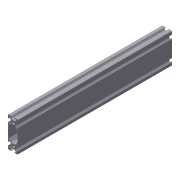
# Autodesk Inventor part: Bosch 20x60
Saved by Autodesk Inventor 2013 (Build 170138000, 138)
## iProperties
Created: 2011-07-21
Part Number: Bosch 20x60
Material: Aluminum-6061
Document SubType Name: Modeling
Designer: Dan Niemitalo
Mass: 296.662 g
Surface Area: 1227.79 cm^2
Volume: 109.469 cm^3
Density: 2.71 g/cm^3
Author: Dan Niemitalo
Autodesk Inventor part; units mm, degrees
ref_plane "YZ Plane" through (0, 0, 0) normal (1, 0, 0) x (0, 1, 0)
ref_plane "XZ Plane" through (0, 0, 0) normal (0, 1, 0) x (-1, 0, 0)
ref_plane "XY Plane" through (0, 0, 0) normal (0, 0, 1) x (1, 0, 0)
sketch "2060" plane through (0, 0, 0) normal (0, 0, 1) x (1, 0, 0)
  line L0 (-1.4693, -31.5636) -> (-0.9592, -32.4471)
  arc A0 (-0.9592, -32.6471) -> (-0.9592, -32.4471) centre (-1.1324, -32.5471) ccw
  line L1 (-0.9592, -32.6471) -> (-1.4693, -33.5306)
  arc A1 (-1.4693, -33.5306) -> (-1.4961, -33.6306) centre (-1.2961, -33.6306) ccw
  line L2 (-1.4961, -33.6306) -> (-1.4961, -35.6543)
  line L3 (0.6358, -33.8094) -> (0.0893, -34.461)
  arc A2 (0.0893, -34.461) -> (1.169, -35.5393) centre (3.0789, -32.5471) ccw
  line L4 (1.169, -35.5393) -> (1.8208, -34.9924)
  arc A3 (2.1254, -37.0471) -> (2.2254, -37.0203) centre (2.1254, -36.8471) ccw
  line L5 (2.2254, -37.0203) -> (2.9789, -36.5852)
  arc A4 (3.1789, -36.5852) -> (2.9789, -36.5852) centre (3.0789, -36.7584) ccw
  line L6 (3.1789, -36.5852) -> (3.9325, -37.0203)
  arc A5 (3.9325, -37.0203) -> (4.0325, -37.0471) centre (4.0325, -36.8471) ccw
  line L7 (4.0325, -37.0471) -> (6.3112, -37.0471)
  line L8 (7.6539, -35.6543) -> (7.6539, -33.6306)
  arc A6 (4.9928, -35.5368) -> (6.0711, -34.457) centre (3.0789, -32.5471) ccw
  line L9 (6.0711, -34.457) -> (5.5242, -33.8053)
  line L10 (4.3413, -34.9902) -> (4.9928, -35.5368)
  arc A7 (7.6539, -35.6543) -> (7.8004, -36.0079) centre (8.1539, -35.6543) ccw
  line L11 (4.9889, -29.5549) -> (4.3371, -30.1018)
  line L12 (1.8166, -30.1039) -> (1.165, -29.5575)
  arc A8 (6.0686, -30.6332) -> (4.9889, -29.5549) centre (3.0789, -32.5471) ccw
  arc A9 (1.165, -29.5575) -> (0.0868, -30.6372) centre (3.0789, -32.5471) ccw
  line L13 (0.0868, -30.6372) -> (0.6336, -31.2889)
  line L14 (5.5242, -31.2889) -> (6.0686, -30.6332)
  arc A10 (0.6336, -31.2889) -> (0.6358, -33.8094) centre (3.0789, -32.5471) ccw
  arc A11 (5.5242, -33.8053) -> (5.5242, -31.2889) centre (3.0789, -32.5471) ccw
  arc A12 (1.8208, -34.9924) -> (4.3413, -34.9902) centre (3.0789, -32.5471) ccw
  arc A13 (4.3371, -30.1018) -> (1.8166, -30.1039) centre (3.0789, -32.5471) ccw
  line L15 (7.6539, -31.4636) -> (7.6539, -29.4399)
  line L16 (7.1171, -32.4471) -> (7.6271, -31.5636)
  arc A14 (7.1171, -32.4471) -> (7.1171, -32.6471) centre (7.2903, -32.5471) ccw
  arc A15 (7.6539, -33.6306) -> (7.6271, -33.5306) centre (7.4539, -33.6306) ccw
  line L17 (7.6271, -33.5306) -> (7.1171, -32.6471)
  arc A16 (7.6271, -31.5636) -> (7.6539, -31.4636) centre (7.4539, -31.4636) ccw
  arc A17 (2.9789, -28.509) -> (3.1789, -28.509) centre (3.0789, -28.3358) ccw
  line L18 (3.1789, -28.509) -> (3.9325, -28.0739)
  line L19 (2.2254, -28.0739) -> (2.9789, -28.509)
  arc A18 (7.8004, -29.0863) -> (7.6539, -29.4399) centre (8.1539, -29.4399) ccw
  line L20 (7.8004, -29.0863) -> (10.1932, -26.6935)
  arc A19 (11.5789, -29.0471) -> (12.0789, -29.5471) centre (12.0789, -29.0471) ccw
  arc A20 (12.3789, -29.5471) -> (12.5789, -29.3471) centre (12.3789, -29.3471) ccw
  line L21 (12.5789, -29.3471) -> (12.5789, -29.2471)
  arc A21 (12.7789, -29.0471) -> (12.5789, -29.2471) centre (12.7789, -29.2471) ccw
  line L22 (12.7789, -29.0471) -> (12.8789, -29.0471)
  line L23 (11.5789, -27.0471) -> (11.5789, -29.0471)
  arc A22 (12.8789, -29.0471) -> (13.0789, -28.8471) centre (12.8789, -28.8471) ccw
  line L24 (12.0789, -29.5471) -> (12.3789, -29.5471)
  arc A23 (-5.4211, -36.0471) -> (-5.9211, -35.5471) centre (-5.9211, -36.0471) ccw
  line L25 (-5.9211, -35.5471) -> (-6.2211, -35.5471)
  line L26 (-6.6211, -36.0971) -> (-6.7211, -36.0971)
  line L27 (-6.4211, -35.7471) -> (-6.4211, -35.8971)
  arc A24 (-6.6211, -36.0971) -> (-6.4211, -35.8971) centre (-6.6211, -35.8971) ccw
  arc A25 (-6.7211, -36.0971) -> (-6.9211, -36.2971) centre (-6.7211, -36.2971) ccw
  arc A26 (-6.2211, -35.5471) -> (-6.4211, -35.7471) centre (-6.2211, -35.7471) ccw
  arc A27 (-1.4961, -31.4636) -> (-1.4693, -31.5636) centre (-1.2961, -31.4636) ccw
  line L28 (-1.4961, -29.4399) -> (-1.4961, -31.4636)
  arc A28 (-1.4961, -29.4399) -> (-1.6425, -29.0863) centre (-1.9961, -29.4399) ccw
  line L29 (-6.2211, -29.5471) -> (-5.9211, -29.5471)
  arc A29 (-5.9211, -29.5471) -> (-5.4211, -29.0471) centre (-5.9211, -29.0471) ccw
  arc A30 (-6.4211, -29.3471) -> (-6.2211, -29.5471) centre (-6.2211, -29.3471) ccw
  line L30 (-6.4211, -29.1971) -> (-6.4211, -29.3471)
  arc A31 (-6.4211, -29.1971) -> (-6.6211, -28.9971) centre (-6.6211, -29.1971) ccw
  line L31 (-6.7211, -28.9971) -> (-6.6211, -28.9971)
  arc A32 (-6.9211, -28.7971) -> (-6.7211, -28.9971) centre (-6.7211, -28.7971) ccw
  line L32 (-4.9211, -26.5471) -> (-4.3888, -26.5471)
  line L33 (-4.0353, -26.6935) -> (-1.6425, -29.0863)
  line L34 (-5.4211, -29.0471) -> (-5.4211, -27.0471)
  arc A33 (-4.0353, -26.6935) -> (-4.3888, -26.5471) centre (-4.3888, -27.0471) ccw
  line L35 (11.5789, 3.9087) -> (11.5789, 1.9587)
  arc A34 (11.0789, 1.4587) -> (11.5789, 1.9587) centre (11.0789, 1.9587) ccw
  line L36 (11.0789, 1.4587) -> (10.3467, 1.4587)
  arc A35 (9.9932, 1.6051) -> (10.3467, 1.4587) centre (10.3467, 1.9587) ccw
  line L37 (11.5789, -2.102) -> (6.6647, 2.8122)
  line L38 (9.9932, 1.6051) -> (7.8004, 3.7979)
  arc A36 (6.6647, 2.8122) -> (6.3112, 2.9587) centre (6.3112, 2.4587) ccw
  line L39 (6.3112, 2.9587) -> (4.0325, 2.9587)
  arc A37 (3.9325, 2.9855) -> (4.0325, 2.9587) centre (4.0325, 3.1587) ccw
  line L40 (3.9325, 2.9855) -> (3.1789, 3.4206)
  arc A38 (3.1789, 3.4206) -> (2.9789, 3.4206) centre (3.0789, 3.2474) ccw
  line L41 (2.9789, 3.4206) -> (2.2254, 2.9855)
  arc A39 (2.1254, 2.9587) -> (2.2254, 2.9855) centre (2.1254, 3.1587) ccw
  arc A40 (12.0789, 4.4087) -> (11.5789, 3.9087) centre (12.0789, 3.9087) ccw
  line L42 (12.3789, 4.4087) -> (12.0789, 4.4087)
  line L43 (12.8789, 3.9087) -> (12.7789, 3.9087)
  line L44 (12.5789, 4.1087) -> (12.5789, 4.2087)
  arc A41 (12.5789, 4.1087) -> (12.7789, 3.9087) centre (12.7789, 4.1087) ccw
  arc A42 (12.5789, 4.2087) -> (12.3789, 4.4087) centre (12.3789, 4.2087) ccw
  arc A43 (13.0789, 3.7087) -> (12.8789, 3.9087) centre (12.8789, 3.7087) ccw
  line L45 (4.3371, 5.0134) -> (4.966, 4.511)
  arc A44 (4.966, 4.511) -> (6.0267, 5.5716) centre (3.0789, 7.4587) ccw
  line L46 (6.0267, 5.5716) -> (5.5242, 6.2005)
  arc A45 (7.6539, 4.1515) -> (7.8004, 3.7979) centre (8.1539, 4.1515) ccw
  line L47 (7.6539, 4.1515) -> (7.6539, 6.6301)
  line L48 (-5.4211, 1.9587) -> (-5.4211, 3.9087)
  arc A46 (-5.4211, 1.9587) -> (-4.9211, 1.4587) centre (-4.9211, 1.9587) ccw
  line L49 (-4.1888, 1.4587) -> (-4.9211, 1.4587)
  arc A47 (-4.1888, 1.4587) -> (-3.8353, 1.6051) centre (-4.1888, 1.9587) ccw
  arc A48 (-1.6425, 3.7979) -> (-1.4961, 4.1515) centre (-1.9961, 4.1515) ccw
  line L50 (-1.6425, 3.7979) -> (-3.8353, 1.6051)
  arc A49 (-0.1533, 2.9587) -> (-0.5068, 2.8122) centre (-0.1533, 2.4587) ccw
  line L51 (-0.5068, 2.8122) -> (-5.4211, -2.102)
  arc A50 (-4.9211, -26.5471) -> (-5.4211, -27.0471) centre (-4.9211, -27.0471) ccw
  arc A51 (-0.5068, -27.9006) -> (-0.1533, -28.0471) centre (-0.1533, -27.5471) ccw
  line L52 (-0.1533, -28.0471) -> (2.1254, -28.0471)
  arc A52 (2.2254, -28.0739) -> (2.1254, -28.0471) centre (2.1254, -28.2471) ccw
  line L53 (-5.4211, -22.9864) -> (-0.5068, -27.9006)
  arc A53 (4.0325, -28.0471) -> (3.9325, -28.0739) centre (4.0325, -28.2471) ccw
  line L54 (4.0325, -28.0471) -> (6.3112, -28.0471)
  arc A54 (6.3112, -28.0471) -> (6.6647, -27.9006) centre (6.3112, -27.5471) ccw
  arc A55 (10.5467, -26.5471) -> (10.1932, -26.6935) centre (10.5467, -27.0471) ccw
  line L55 (10.5467, -26.5471) -> (11.0789, -26.5471)
  arc A56 (11.5789, -27.0471) -> (11.0789, -26.5471) centre (11.0789, -27.0471) ccw
  line L56 (6.6647, -27.9006) -> (11.5789, -22.9864)
  line L57 (-6.9211, 3.7087) -> (-6.9211, -28.7971)
  line L58 (13.0789, -28.8471) -> (13.0789, 3.7087)
  line L59 (11.5789, -22.9864) -> (11.5789, -2.102)
  line L60 (-5.4211, -2.102) -> (-5.4211, -22.9864)
  arc A57 (-6.7211, 3.9087) -> (-6.9211, 3.7087) centre (-6.7211, 3.7087) ccw
  line L61 (-6.6211, 3.9087) -> (-6.7211, 3.9087)
  arc A58 (-6.6211, 3.9087) -> (-6.4211, 4.1087) centre (-6.6211, 4.1087) ccw
  arc A59 (-5.4211, 3.9087) -> (-5.9211, 4.4087) centre (-5.9211, 3.9087) ccw
  line L62 (-5.9211, 4.4087) -> (-6.2211, 4.4087)
  arc A60 (-6.2211, 4.4087) -> (-6.4211, 4.2087) centre (-6.2211, 4.2087) ccw
  line L63 (-6.4211, 4.2087) -> (-6.4211, 4.1087)
  line L64 (5.5242, 8.7169) -> (6.0267, 9.3457)
  line L65 (4.966, 10.4064) -> (4.3371, 9.904)
  arc A61 (6.0267, 9.3457) -> (4.966, 10.4064) centre (3.0789, 7.4587) ccw
  arc A62 (11.5789, 10.9087) -> (12.0789, 10.4087) centre (12.0789, 10.9087) ccw
  line L66 (12.0789, 10.4087) -> (12.3789, 10.4087)
  line L67 (12.7789, 10.9087) -> (12.8789, 10.9087)
  line L68 (12.5789, 10.6087) -> (12.5789, 10.7087)
  arc A63 (12.7789, 10.9087) -> (12.5789, 10.7087) centre (12.7789, 10.7087) ccw
  arc A64 (12.3789, 10.4087) -> (12.5789, 10.6087) centre (12.3789, 10.6087) ccw
  arc A65 (12.8789, 10.9087) -> (13.0789, 11.1087) centre (12.8789, 11.1087) ccw
  arc A66 (5.5242, 6.2005) -> (5.5242, 8.7169) centre (3.0789, 7.4587) ccw
  arc A67 (1.8208, 5.0134) -> (4.3371, 5.0134) centre (3.0789, 7.4587) ccw
  line L69 (1.1919, 4.511) -> (1.8208, 5.0134)
  line L70 (2.1254, 2.9587) -> (-0.1533, 2.9587)
  arc A68 (0.1312, 5.5716) -> (1.1919, 4.511) centre (3.0789, 7.4587) ccw
  arc A69 (4.3371, 9.904) -> (1.8208, 9.904) centre (3.0789, 7.4587) ccw
  line L71 (0.6336, 6.2005) -> (0.1312, 5.5716)
  arc A70 (0.6336, 8.7169) -> (0.6336, 6.2005) centre (3.0789, 7.4587) ccw
  line L72 (1.8208, 9.904) -> (1.1919, 10.4064)
  line L73 (0.1312, 9.3457) -> (0.6336, 8.7169)
  arc A71 (1.1919, 10.4064) -> (0.1312, 9.3457) centre (3.0789, 7.4587) ccw
  arc A72 (7.6539, 6.6301) -> (7.6271, 6.7301) centre (7.4539, 6.6301) ccw
  line L74 (7.6271, 6.7301) -> (7.2209, 7.4337)
  arc A73 (7.2209, 7.6337) -> (7.2209, 7.4337) centre (7.3941, 7.5337) ccw
  line L75 (7.2209, 7.6337) -> (7.6271, 8.3373)
  arc A74 (7.6271, 8.3373) -> (7.6539, 8.4373) centre (7.4539, 8.4373) ccw
  line L76 (7.6539, 8.4373) -> (7.6539, 10.7659)
  arc A75 (6.3112, 11.9529) -> (6.6647, 12.0994) centre (6.3112, 12.4529) ccw
  arc A76 (-1.4961, 10.7659) -> (-1.6425, 11.1195) centre (-1.9961, 10.7659) ccw
  line L77 (-1.4961, 10.7659) -> (-1.4961, 8.4373)
  line L78 (6.3112, 11.9529) -> (4.0325, 11.9529)
  arc A77 (4.0325, 11.9529) -> (3.9325, 11.9261) centre (4.0325, 11.7529) ccw
  line L79 (3.9325, 11.9261) -> (3.1381, 11.4675)
  arc A78 (3.0197, 11.4675) -> (3.1381, 11.4675) centre (3.0789, 11.57) ccw
  arc A79 (2.2254, 11.9261) -> (2.1254, 11.9529) centre (2.1254, 11.7529) ccw
  line L80 (3.0197, 11.4675) -> (2.2254, 11.9261)
  line L81 (2.1254, 11.9529) -> (-0.1533, 11.9529)
  line L82 (-6.7211, 10.9087) -> (-6.6211, 10.9087)
  arc A80 (-6.4211, 10.7087) -> (-6.6211, 10.9087) centre (-6.6211, 10.7087) ccw
  line L83 (-6.4211, 10.7087) -> (-6.4211, 10.6087)
  line L84 (-6.2211, 10.4087) -> (-5.9211, 10.4087)
  arc A81 (-5.9211, 10.4087) -> (-5.4211, 10.9087) centre (-5.9211, 10.9087) ccw
  arc A82 (-6.4211, 10.6087) -> (-6.2211, 10.4087) centre (-6.2211, 10.6087) ccw
  arc A83 (-1.4961, 8.4373) -> (-1.4693, 8.3373) centre (-1.2961, 8.4373) ccw
  line L85 (-1.4693, 8.3373) -> (-1.063, 7.6337)
  arc A84 (-1.063, 7.4337) -> (-1.063, 7.6337) centre (-1.2363, 7.5337) ccw
  line L86 (-1.063, 7.4337) -> (-1.4693, 6.7301)
  arc A85 (-1.4693, 6.7301) -> (-1.4961, 6.6301) centre (-1.2961, 6.6301) ccw
  line L87 (-1.4961, 6.6301) -> (-1.4961, 4.1515)
  line L88 (9.0789, 15.4529) -> (9.0789, 14.7207)
  arc A86 (8.9325, 14.3671) -> (9.0789, 14.7207) centre (8.5789, 14.7207) ccw
  line L89 (8.9325, 14.3671) -> (6.6647, 12.0994)
  arc A87 (10.3467, 13.4587) -> (9.9932, 13.3122) centre (10.3467, 12.9587) ccw
  arc A88 (11.5789, 12.9587) -> (11.0789, 13.4587) centre (11.0789, 12.9587) ccw
  line L90 (7.8004, 11.1195) -> (9.9932, 13.3122)
  arc A89 (7.8004, 11.1195) -> (7.6539, 10.7659) centre (8.1539, 10.7659) ccw
  line L91 (13.0789, 11.1087) -> (13.0789, 15.9529)
  line L92 (11.5789, 12.9587) -> (11.5789, 10.9087)
  line L93 (10.3467, 13.4587) -> (11.0789, 13.4587)
  arc A90 (9.0789, 15.4529) -> (8.5789, 15.9529) centre (8.5789, 15.4529) ccw
  arc A91 (13.0789, 15.9529) -> (11.5789, 17.4529) centre (11.5789, 15.9529) ccw
  line L94 (11.5789, 17.4529) -> (6.8289, 17.4529)
  line L95 (6.5789, 15.9529) -> (8.5789, 15.9529)
  arc A92 (6.0789, 16.4529) -> (6.5789, 15.9529) centre (6.5789, 16.4529) ccw
  line L96 (6.6289, 17.2529) -> (6.6289, 17.1529)
  line L97 (6.0789, 16.7529) -> (6.0789, 16.4529)
  arc A93 (6.4289, 16.9529) -> (6.6289, 17.1529) centre (6.4289, 17.1529) ccw
  arc A94 (6.8289, 17.4529) -> (6.6289, 17.2529) centre (6.8289, 17.2529) ccw
  arc A95 (6.2789, 16.9529) -> (6.0789, 16.7529) centre (6.2789, 16.7529) ccw
  line L98 (6.4289, 16.9529) -> (6.2789, 16.9529)
  arc A96 (-0.4211, 15.9529) -> (0.0789, 16.4529) centre (-0.4211, 16.4529) ccw
  line L99 (-0.4711, 17.1529) -> (-0.4711, 17.2529)
  line L100 (-0.1211, 16.9529) -> (-0.2711, 16.9529)
  line L101 (0.0789, 16.4529) -> (0.0789, 16.7529)
  arc A97 (-0.4711, 17.1529) -> (-0.2711, 16.9529) centre (-0.2711, 17.1529) ccw
  arc A98 (-0.4711, 17.2529) -> (-0.6711, 17.4529) centre (-0.6711, 17.2529) ccw
  arc A99 (0.0789, 16.7529) -> (-0.1211, 16.9529) centre (-0.1211, 16.7529) ccw
  line L102 (-2.4211, 15.9529) -> (-0.4211, 15.9529)
  line L103 (-4.9211, 13.4587) -> (-4.1888, 13.4587)
  arc A100 (-3.8353, 13.3122) -> (-4.1888, 13.4587) centre (-4.1888, 12.9587) ccw
  line L104 (-2.9211, 14.7207) -> (-2.9211, 15.4529)
  arc A101 (-2.9211, 14.7207) -> (-2.7746, 14.3671) centre (-2.4211, 14.7207) ccw
  arc A102 (-2.4211, 15.9529) -> (-2.9211, 15.4529) centre (-2.4211, 15.4529) ccw
  line L105 (-0.6711, 17.4529) -> (-5.4211, 17.4529)
  line L106 (-3.8353, 13.3122) -> (-1.6425, 11.1195)
  line L107 (-0.5068, 12.0994) -> (-2.7746, 14.3671)
  arc A103 (-0.5068, 12.0994) -> (-0.1533, 11.9529) centre (-0.1533, 12.4529) ccw
  arc A104 (-4.9211, 13.4587) -> (-5.4211, 12.9587) centre (-4.9211, 12.9587) ccw
  line L108 (-5.4211, 10.9087) -> (-5.4211, 12.9587)
  arc A105 (-6.9211, 11.1087) -> (-6.7211, 10.9087) centre (-6.7211, 11.1087) ccw
  line L109 (-6.9211, 15.9529) -> (-6.9211, 11.1087)
  arc A106 (-5.4211, 17.4529) -> (-6.9211, 15.9529) centre (-5.4211, 15.9529) ccw
  arc A107 (6.6647, -37.1935) -> (6.3112, -37.0471) centre (6.3112, -37.5471) ccw
  arc A108 (-2.9211, -40.5471) -> (-2.4211, -41.0471) centre (-2.4211, -40.5471) ccw
  line L110 (-2.9211, -40.5471) -> (-2.9211, -39.8149)
  arc A109 (-2.7746, -39.4613) -> (-2.9211, -39.8149) centre (-2.4211, -39.8149) ccw
  line L111 (-2.7746, -39.4613) -> (-0.5068, -37.1935)
  line L112 (-1.6425, -36.0079) -> (-4.0353, -38.4006)
  arc A110 (-1.6425, -36.0079) -> (-1.4961, -35.6543) centre (-1.9961, -35.6543) ccw
  arc A111 (-0.1533, -37.0471) -> (-0.5068, -37.1935) centre (-0.1533, -37.5471) ccw
  line L113 (-0.1533, -37.0471) -> (2.1254, -37.0471)
  line L114 (10.1932, -38.4006) -> (7.8004, -36.0079)
  line L115 (9.0789, -39.8149) -> (9.0789, -40.5471)
  arc A112 (9.0789, -39.8149) -> (8.9325, -39.4613) centre (8.5789, -39.8149) ccw
  line L116 (6.6647, -37.1935) -> (8.9325, -39.4613)
  arc A113 (10.1932, -38.4006) -> (10.5467, -38.5471) centre (10.5467, -38.0471) ccw
  line L117 (11.0789, -38.5471) -> (10.5467, -38.5471)
  arc A114 (11.0789, -38.5471) -> (11.5789, -38.0471) centre (11.0789, -38.0471) ccw
  line L118 (11.5789, -36.0471) -> (11.5789, -38.0471)
  arc A115 (12.0789, -35.5471) -> (11.5789, -36.0471) centre (12.0789, -36.0471) ccw
  line L119 (12.3789, -35.5471) -> (12.0789, -35.5471)
  arc A116 (12.5789, -35.7471) -> (12.3789, -35.5471) centre (12.3789, -35.7471) ccw
  line L120 (12.5789, -35.8471) -> (12.5789, -35.7471)
  arc A117 (12.5789, -35.8471) -> (12.7789, -36.0471) centre (12.7789, -35.8471) ccw
  line L121 (12.8789, -36.0471) -> (12.7789, -36.0471)
  arc A118 (13.0789, -36.2471) -> (12.8789, -36.0471) centre (12.8789, -36.2471) ccw
  line L122 (13.0789, -41.0471) -> (13.0789, -36.2471)
  arc A119 (-4.3888, -38.5471) -> (-4.0353, -38.4006) centre (-4.3888, -38.0471) ccw
  line L123 (-4.3888, -38.5471) -> (-4.9211, -38.5471)
  arc A120 (-6.9211, -41.0471) -> (-5.4211, -42.5471) centre (-5.4211, -41.0471) ccw
  arc A121 (-5.4211, -38.0471) -> (-4.9211, -38.5471) centre (-4.9211, -38.0471) ccw
  line L124 (-6.9211, -36.2971) -> (-6.9211, -41.0471)
  line L125 (-5.4211, -38.0471) -> (-5.4211, -36.0471)
  arc A122 (0.0789, -41.5471) -> (-0.4211, -41.0471) centre (-0.4211, -41.5471) ccw
  line L126 (0.0789, -41.8471) -> (0.0789, -41.5471)
  arc A123 (-0.1211, -42.0471) -> (0.0789, -41.8471) centre (-0.1211, -41.8471) ccw
  line L127 (-0.2711, -42.0471) -> (-0.1211, -42.0471)
  arc A124 (-0.2711, -42.0471) -> (-0.4711, -42.2471) centre (-0.2711, -42.2471) ccw
  line L128 (-0.4711, -42.3471) -> (-0.4711, -42.2471)
  arc A125 (-0.6711, -42.5471) -> (-0.4711, -42.3471) centre (-0.6711, -42.3471) ccw
  line L129 (-5.4211, -42.5471) -> (-0.6711, -42.5471)
  line L130 (-0.4211, -41.0471) -> (-2.4211, -41.0471)
  line L131 (6.6289, -42.2471) -> (6.6289, -42.3471)
  line L132 (6.2789, -42.0471) -> (6.4289, -42.0471)
  line L133 (6.0789, -41.5471) -> (6.0789, -41.8471)
  arc A126 (6.6289, -42.2471) -> (6.4289, -42.0471) centre (6.4289, -42.2471) ccw
  arc A127 (6.6289, -42.3471) -> (6.8289, -42.5471) centre (6.8289, -42.3471) ccw
  arc A128 (6.0789, -41.8471) -> (6.2789, -42.0471) centre (6.2789, -41.8471) ccw
  arc A129 (6.5789, -41.0471) -> (6.0789, -41.5471) centre (6.5789, -41.5471) ccw
  arc A130 (11.5789, -42.5471) -> (13.0789, -41.0471) centre (11.5789, -41.0471) ccw
  line L134 (6.8289, -42.5471) -> (11.5789, -42.5471)
  line L135 (8.5789, -41.0471) -> (6.5789, -41.0471)
  arc A131 (8.5789, -41.0471) -> (9.0789, -40.5471) centre (8.5789, -40.5471) ccw
  point P0 (3.0789, -12.5479)
sketch "Sketch1" plane through (0, 0, 0) normal (0, 0, 1) x (1, 0, 0)
  line L0 (-4.5482, -19.0194) -> (-4.0381, -19.9029)
  arc A0 (-4.0381, -20.1029) -> (-4.0381, -19.9029) centre (-4.2113, -20.0029) ccw
  line L1 (-4.0381, -20.1029) -> (-4.5482, -20.9864)
  arc A1 (-4.5482, -20.9864) -> (-4.575, -21.0864) centre (-4.375, -21.0864) ccw
  line L2 (-4.575, -21.0864) -> (-4.575, -23.1101)
  line L3 (-2.4431, -21.2652) -> (-2.9897, -21.9168)
  arc A2 (-2.9897, -21.9168) -> (-1.9099, -22.9951) centre (0, -20.0029) ccw
  line L4 (-1.9099, -22.9951) -> (-1.2582, -22.4482)
  arc A3 (-0.9536, -24.5029) -> (-0.8536, -24.4761) centre (-0.9536, -24.3029) ccw
  line L5 (-0.8536, -24.4761) -> (-0.1, -24.041)
  arc A4 (0.1, -24.041) -> (-0.1, -24.041) centre (0, -24.2142) ccw
  line L6 (0.1, -24.041) -> (0.8536, -24.4761)
  arc A5 (0.8536, -24.4761) -> (0.9536, -24.5029) centre (0.9536, -24.3029) ccw
  line L7 (0.9536, -24.5029) -> (3.2322, -24.5029)
  line L8 (4.575, -23.1101) -> (4.575, -21.0864)
  arc A6 (1.9139, -22.9926) -> (2.9922, -21.9128) centre (0, -20.0029) ccw
  line L9 (2.9922, -21.9128) -> (2.4453, -21.2611)
  line L10 (1.2623, -22.446) -> (1.9139, -22.9926)
  arc A7 (4.575, -23.1101) -> (4.7214, -23.4637) centre (5.075, -23.1101) ccw
  line L11 (1.9099, -17.0107) -> (1.2582, -17.5576)
  line L12 (-1.2623, -17.5597) -> (-1.9139, -17.0133)
  arc A8 (2.9896, -18.089) -> (1.9099, -17.0107) centre (0, -20.0029) ccw
  arc A9 (-1.9139, -17.0133) -> (-2.9922, -18.093) centre (0, -20.0029) ccw
  line L13 (-2.9922, -18.093) -> (-2.4453, -18.7447)
  line L14 (2.4453, -18.7447) -> (2.9896, -18.089)
  arc A10 (-2.4453, -18.7447) -> (-2.4431, -21.2652) centre (0, -20.0029) ccw
  arc A11 (2.4453, -21.2611) -> (2.4453, -18.7447) centre (0, -20.0029) ccw
  arc A12 (-1.2582, -22.4482) -> (1.2623, -22.446) centre (0, -20.0029) ccw
  arc A13 (1.2582, -17.5576) -> (-1.2623, -17.5597) centre (0, -20.0029) ccw
  line L15 (4.575, -18.9194) -> (4.575, -16.8957)
  line L16 (4.0381, -19.9029) -> (4.5482, -19.0194)
  arc A14 (4.0381, -19.9029) -> (4.0381, -20.1029) centre (4.2113, -20.0029) ccw
  arc A15 (4.575, -21.0864) -> (4.5482, -20.9864) centre (4.375, -21.0864) ccw
  line L17 (4.5482, -20.9864) -> (4.0381, -20.1029)
  arc A16 (4.5482, -19.0194) -> (4.575, -18.9194) centre (4.375, -18.9194) ccw
  arc A17 (-0.1, -15.9648) -> (0.1, -15.9648) centre (0, -15.7916) ccw
  line L18 (0.1, -15.9648) -> (0.8536, -15.5297)
  line L19 (-0.8536, -15.5297) -> (-0.1, -15.9648)
  arc A18 (4.7214, -16.5421) -> (4.575, -16.8957) centre (5.075, -16.8957) ccw
  line L20 (4.7214, -16.5421) -> (7.1142, -14.1493)
  arc A19 (8.5, -16.5029) -> (9, -17.0029) centre (9, -16.5029) ccw
  arc A20 (9.3, -17.0029) -> (9.5, -16.8029) centre (9.3, -16.8029) ccw
  line L21 (9.5, -16.8029) -> (9.5, -16.7029)
  arc A21 (9.7, -16.5029) -> (9.5, -16.7029) centre (9.7, -16.7029) ccw
  line L22 (9.7, -16.5029) -> (9.8, -16.5029)
  line L23 (8.5, -14.5029) -> (8.5, -16.5029)
  arc A22 (9.8, -16.5029) -> (10, -16.3029) centre (9.8, -16.3029) ccw
  line L24 (9, -17.0029) -> (9.3, -17.0029)
  arc A23 (-8.5, -23.5029) -> (-9, -23.0029) centre (-9, -23.5029) ccw
  line L25 (-9, -23.0029) -> (-9.3, -23.0029)
  line L26 (-9.7, -23.5529) -> (-9.8, -23.5529)
  line L27 (-9.5, -23.2029) -> (-9.5, -23.3529)
  arc A24 (-9.7, -23.5529) -> (-9.5, -23.3529) centre (-9.7, -23.3529) ccw
  arc A25 (-9.8, -23.5529) -> (-10, -23.7529) centre (-9.8, -23.7529) ccw
  arc A26 (-9.3, -23.0029) -> (-9.5, -23.2029) centre (-9.3, -23.2029) ccw
  arc A27 (-4.575, -18.9194) -> (-4.5482, -19.0194) centre (-4.375, -18.9194) ccw
  line L28 (-4.575, -16.8957) -> (-4.575, -18.9194)
  arc A28 (-4.575, -16.8957) -> (-4.7214, -16.5421) centre (-5.075, -16.8957) ccw
  line L29 (-9.3, -17.0029) -> (-9, -17.0029)
  arc A29 (-9, -17.0029) -> (-8.5, -16.5029) centre (-9, -16.5029) ccw
  arc A30 (-9.5, -16.8029) -> (-9.3, -17.0029) centre (-9.3, -16.8029) ccw
  line L30 (-9.5, -16.6529) -> (-9.5, -16.8029)
  arc A31 (-9.5, -16.6529) -> (-9.7, -16.4529) centre (-9.7, -16.6529) ccw
  line L31 (-9.8, -16.4529) -> (-9.7, -16.4529)
  arc A32 (-10, -16.2529) -> (-9.8, -16.4529) centre (-9.8, -16.2529) ccw
  line L32 (-8, -14.0029) -> (-7.4678, -14.0029)
  line L33 (-7.1142, -14.1493) -> (-4.7214, -16.5421)
  line L34 (-8.5, -16.5029) -> (-8.5, -14.5029)
  arc A33 (-7.1142, -14.1493) -> (-7.4678, -14.0029) centre (-7.4678, -14.5029) ccw
  line L35 (8.5, 16.4529) -> (8.5, 14.5029)
  arc A34 (8, 14.0029) -> (8.5, 14.5029) centre (8, 14.5029) ccw
  line L36 (8, 14.0029) -> (7.2678, 14.0029)
  arc A35 (6.9142, 14.1493) -> (7.2678, 14.0029) centre (7.2678, 14.5029) ccw
  line L37 (8.5, 10.4422) -> (3.5858, 15.3564)
  line L38 (6.9142, 14.1493) -> (4.7214, 16.3421)
  arc A36 (3.5858, 15.3564) -> (3.2322, 15.5029) centre (3.2322, 15.0029) ccw
  line L39 (3.2322, 15.5029) -> (0.9536, 15.5029)
  arc A37 (0.8536, 15.5297) -> (0.9536, 15.5029) centre (0.9536, 15.7029) ccw
  line L40 (0.8536, 15.5297) -> (0.1, 15.9648)
  arc A38 (0.1, 15.9648) -> (-0.1, 15.9648) centre (0, 15.7916) ccw
  line L41 (-0.1, 15.9648) -> (-0.8536, 15.5297)
  arc A39 (-0.9536, 15.5029) -> (-0.8536, 15.5297) centre (-0.9536, 15.7029) ccw
  arc A40 (9, 16.9529) -> (8.5, 16.4529) centre (9, 16.4529) ccw
  line L42 (9.3, 16.9529) -> (9, 16.9529)
  line L43 (9.8, 16.4529) -> (9.7, 16.4529)
  line L44 (9.5, 16.6529) -> (9.5, 16.7529)
  arc A41 (9.5, 16.6529) -> (9.7, 16.4529) centre (9.7, 16.6529) ccw
  arc A42 (9.5, 16.7529) -> (9.3, 16.9529) centre (9.3, 16.7529) ccw
  arc A43 (10, 16.2529) -> (9.8, 16.4529) centre (9.8, 16.2529) ccw
  line L45 (1.2582, 17.5576) -> (1.8871, 17.0552)
  arc A44 (1.8871, 17.0552) -> (2.9477, 18.1158) centre (0, 20.0029) ccw
  line L46 (2.9477, 18.1158) -> (2.4453, 18.7447)
  arc A45 (4.575, 16.6957) -> (4.7214, 16.3421) centre (5.075, 16.6957) ccw
  line L47 (4.575, 16.6957) -> (4.575, 19.1743)
  line L48 (-8.5, 14.5029) -> (-8.5, 16.4529)
  arc A46 (-8.5, 14.5029) -> (-8, 14.0029) centre (-8, 14.5029) ccw
  line L49 (-7.2678, 14.0029) -> (-8, 14.0029)
  arc A47 (-7.2678, 14.0029) -> (-6.9142, 14.1493) centre (-7.2678, 14.5029) ccw
  arc A48 (-4.7214, 16.3421) -> (-4.575, 16.6957) centre (-5.075, 16.6957) ccw
  line L50 (-4.7214, 16.3421) -> (-6.9142, 14.1493)
  arc A49 (-3.2322, 15.5029) -> (-3.5858, 15.3564) centre (-3.2322, 15.0029) ccw
  line L51 (-3.5858, 15.3564) -> (-8.5, 10.4422)
  arc A50 (-8, -14.0029) -> (-8.5, -14.5029) centre (-8, -14.5029) ccw
  arc A51 (-3.5858, -15.3564) -> (-3.2322, -15.5029) centre (-3.2322, -15.0029) ccw
  line L52 (-3.2322, -15.5029) -> (-0.9536, -15.5029)
  arc A52 (-0.8536, -15.5297) -> (-0.9536, -15.5029) centre (-0.9536, -15.7029) ccw
  line L53 (-8.5, -10.4422) -> (-3.5858, -15.3564)
  arc A53 (0.9536, -15.5029) -> (0.8536, -15.5297) centre (0.9536, -15.7029) ccw
  line L54 (0.9536, -15.5029) -> (3.2322, -15.5029)
  arc A54 (3.2322, -15.5029) -> (3.5858, -15.3564) centre (3.2322, -15.0029) ccw
  arc A55 (7.4678, -14.0029) -> (7.1142, -14.1493) centre (7.4678, -14.5029) ccw
  line L55 (7.4678, -14.0029) -> (8, -14.0029)
  arc A56 (8.5, -14.5029) -> (8, -14.0029) centre (8, -14.5029) ccw
  line L56 (3.5858, -15.3564) -> (8.5, -10.4422)
  line L57 (-10, 16.2529) -> (-10, -16.2529)
  line L58 (10, -16.3029) -> (10, 16.2529)
  line L59 (8.5, -10.4422) -> (8.5, 10.4422)
  line L60 (-8.5, 10.4422) -> (-8.5, -10.4422)
  arc A57 (-9.8, 16.4529) -> (-10, 16.2529) centre (-9.8, 16.2529) ccw
  line L61 (-9.7, 16.4529) -> (-9.8, 16.4529)
  arc A58 (-9.7, 16.4529) -> (-9.5, 16.6529) centre (-9.7, 16.6529) ccw
  arc A59 (-8.5, 16.4529) -> (-9, 16.9529) centre (-9, 16.4529) ccw
  line L62 (-9, 16.9529) -> (-9.3, 16.9529)
  arc A60 (-9.3, 16.9529) -> (-9.5, 16.7529) centre (-9.3, 16.7529) ccw
  line L63 (-9.5, 16.7529) -> (-9.5, 16.6529)
  line L64 (2.4453, 21.2611) -> (2.9477, 21.8899)
  line L65 (1.8871, 22.9506) -> (1.2582, 22.4482)
  arc A61 (2.9477, 21.8899) -> (1.8871, 22.9506) centre (0, 20.0029) ccw
  arc A62 (8.5, 23.4529) -> (9, 22.9529) centre (9, 23.4529) ccw
  line L66 (9, 22.9529) -> (9.3, 22.9529)
  line L67 (9.7, 23.4529) -> (9.8, 23.4529)
  line L68 (9.5, 23.1529) -> (9.5, 23.2529)
  arc A63 (9.7, 23.4529) -> (9.5, 23.2529) centre (9.7, 23.2529) ccw
  arc A64 (9.3, 22.9529) -> (9.5, 23.1529) centre (9.3, 23.1529) ccw
  arc A65 (9.8, 23.4529) -> (10, 23.6529) centre (9.8, 23.6529) ccw
  arc A66 (2.4453, 18.7447) -> (2.4453, 21.2611) centre (0, 20.0029) ccw
  arc A67 (-1.2582, 17.5576) -> (1.2582, 17.5576) centre (0, 20.0029) ccw
  line L69 (-1.8871, 17.0552) -> (-1.2582, 17.5576)
  line L70 (-0.9536, 15.5029) -> (-3.2322, 15.5029)
  arc A68 (-2.9477, 18.1158) -> (-1.8871, 17.0552) centre (0, 20.0029) ccw
  arc A69 (1.2582, 22.4482) -> (-1.2582, 22.4482) centre (0, 20.0029) ccw
  line L71 (-2.4453, 18.7447) -> (-2.9477, 18.1158)
  arc A70 (-2.4453, 21.2611) -> (-2.4453, 18.7447) centre (0, 20.0029) ccw
  line L72 (-1.2582, 22.4482) -> (-1.8871, 22.9506)
  line L73 (-2.9477, 21.8899) -> (-2.4453, 21.2611)
  arc A71 (-1.8871, 22.9506) -> (-2.9477, 21.8899) centre (0, 20.0029) ccw
  arc A72 (4.575, 19.1743) -> (4.5482, 19.2743) centre (4.375, 19.1743) ccw
  line L74 (4.5482, 19.2743) -> (4.142, 19.9779)
  arc A73 (4.142, 20.1779) -> (4.142, 19.9779) centre (4.3152, 20.0779) ccw
  line L75 (4.142, 20.1779) -> (4.5482, 20.8815)
  arc A74 (4.5482, 20.8815) -> (4.575, 20.9815) centre (4.375, 20.9815) ccw
  line L76 (4.575, 20.9815) -> (4.575, 23.3101)
  arc A75 (3.2322, 24.4971) -> (3.5858, 24.6436) centre (3.2322, 24.9971) ccw
  arc A76 (-4.575, 23.3101) -> (-4.7214, 23.6637) centre (-5.075, 23.3101) ccw
  line L77 (-4.575, 23.3101) -> (-4.575, 20.9815)
  line L78 (3.2322, 24.4971) -> (0.9536, 24.4971)
  arc A77 (0.9536, 24.4971) -> (0.8536, 24.4703) centre (0.9536, 24.2971) ccw
  line L79 (0.8536, 24.4703) -> (0.0592, 24.0117)
  arc A78 (-0.0592, 24.0117) -> (0.0592, 24.0117) centre (0, 24.1142) ccw
  arc A79 (-0.8536, 24.4703) -> (-0.9536, 24.4971) centre (-0.9536, 24.2971) ccw
  line L80 (-0.0592, 24.0117) -> (-0.8536, 24.4703)
  line L81 (-0.9536, 24.4971) -> (-3.2322, 24.4971)
  line L82 (-9.8, 23.4529) -> (-9.7, 23.4529)
  arc A80 (-9.5, 23.2529) -> (-9.7, 23.4529) centre (-9.7, 23.2529) ccw
  line L83 (-9.5, 23.2529) -> (-9.5, 23.1529)
  line L84 (-9.3, 22.9529) -> (-9, 22.9529)
  arc A81 (-9, 22.9529) -> (-8.5, 23.4529) centre (-9, 23.4529) ccw
  arc A82 (-9.5, 23.1529) -> (-9.3, 22.9529) centre (-9.3, 23.1529) ccw
  arc A83 (-4.575, 20.9815) -> (-4.5482, 20.8815) centre (-4.375, 20.9815) ccw
  line L85 (-4.5482, 20.8815) -> (-4.142, 20.1779)
  arc A84 (-4.142, 19.9779) -> (-4.142, 20.1779) centre (-4.3152, 20.0779) ccw
  line L86 (-4.142, 19.9779) -> (-4.5482, 19.2743)
  arc A85 (-4.5482, 19.2743) -> (-4.575, 19.1743) centre (-4.375, 19.1743) ccw
  line L87 (-4.575, 19.1743) -> (-4.575, 16.6957)
  line L88 (6, 27.9971) -> (6, 27.2649)
  arc A86 (5.8536, 26.9113) -> (6, 27.2649) centre (5.5, 27.2649) ccw
  line L89 (5.8536, 26.9113) -> (3.5858, 24.6436)
  arc A87 (7.2678, 26.0029) -> (6.9142, 25.8564) centre (7.2678, 25.5029) ccw
  arc A88 (8.5, 25.5029) -> (8, 26.0029) centre (8, 25.5029) ccw
  line L90 (4.7214, 23.6637) -> (6.9142, 25.8564)
  arc A89 (4.7214, 23.6637) -> (4.575, 23.3101) centre (5.075, 23.3101) ccw
  line L91 (10, 23.6529) -> (10, 28.4971)
  line L92 (8.5, 25.5029) -> (8.5, 23.4529)
  line L93 (7.2678, 26.0029) -> (8, 26.0029)
  arc A90 (6, 27.9971) -> (5.5, 28.4971) centre (5.5, 27.9971) ccw
  arc A91 (10, 28.4971) -> (8.5, 29.9971) centre (8.5, 28.4971) ccw
  line L94 (8.5, 29.9971) -> (3.75, 29.9971)
  line L95 (3.5, 28.4971) -> (5.5, 28.4971)
  arc A92 (3, 28.9971) -> (3.5, 28.4971) centre (3.5, 28.9971) ccw
  line L96 (3.55, 29.7971) -> (3.55, 29.6971)
  line L97 (3, 29.2971) -> (3, 28.9971)
  arc A93 (3.35, 29.4971) -> (3.55, 29.6971) centre (3.35, 29.6971) ccw
  arc A94 (3.75, 29.9971) -> (3.55, 29.7971) centre (3.75, 29.7971) ccw
  arc A95 (3.2, 29.4971) -> (3, 29.2971) centre (3.2, 29.2971) ccw
  line L98 (3.35, 29.4971) -> (3.2, 29.4971)
  arc A96 (-3.5, 28.4971) -> (-3, 28.9971) centre (-3.5, 28.9971) ccw
  line L99 (-3.55, 29.6971) -> (-3.55, 29.7971)
  line L100 (-3.2, 29.4971) -> (-3.35, 29.4971)
  line L101 (-3, 28.9971) -> (-3, 29.2971)
  arc A97 (-3.55, 29.6971) -> (-3.35, 29.4971) centre (-3.35, 29.6971) ccw
  arc A98 (-3.55, 29.7971) -> (-3.75, 29.9971) centre (-3.75, 29.7971) ccw
  arc A99 (-3, 29.2971) -> (-3.2, 29.4971) centre (-3.2, 29.2971) ccw
  line L102 (-5.5, 28.4971) -> (-3.5, 28.4971)
  line L103 (-8, 26.0029) -> (-7.2678, 26.0029)
  arc A100 (-6.9142, 25.8564) -> (-7.2678, 26.0029) centre (-7.2678, 25.5029) ccw
  line L104 (-6, 27.2649) -> (-6, 27.9971)
  arc A101 (-6, 27.2649) -> (-5.8536, 26.9113) centre (-5.5, 27.2649) ccw
  arc A102 (-5.5, 28.4971) -> (-6, 27.9971) centre (-5.5, 27.9971) ccw
  line L105 (-3.75, 29.9971) -> (-8.5, 29.9971)
  line L106 (-6.9142, 25.8564) -> (-4.7214, 23.6637)
  line L107 (-3.5858, 24.6436) -> (-5.8536, 26.9113)
  arc A103 (-3.5858, 24.6436) -> (-3.2322, 24.4971) centre (-3.2322, 24.9971) ccw
  arc A104 (-8, 26.0029) -> (-8.5, 25.5029) centre (-8, 25.5029) ccw
  line L108 (-8.5, 23.4529) -> (-8.5, 25.5029)
  arc A105 (-10, 23.6529) -> (-9.8, 23.4529) centre (-9.8, 23.6529) ccw
  line L109 (-10, 28.4971) -> (-10, 23.6529)
  arc A106 (-8.5, 29.9971) -> (-10, 28.4971) centre (-8.5, 28.4971) ccw
  arc A107 (3.5858, -24.6493) -> (3.2322, -24.5029) centre (3.2322, -25.0029) ccw
  arc A108 (-6, -28.0029) -> (-5.5, -28.5029) centre (-5.5, -28.0029) ccw
  line L110 (-6, -28.0029) -> (-6, -27.2707)
  arc A109 (-5.8536, -26.9171) -> (-6, -27.2707) centre (-5.5, -27.2707) ccw
  line L111 (-5.8536, -26.9171) -> (-3.5858, -24.6493)
  line L112 (-4.7214, -23.4637) -> (-7.1142, -25.8564)
  arc A110 (-4.7214, -23.4637) -> (-4.575, -23.1101) centre (-5.075, -23.1101) ccw
  arc A111 (-3.2322, -24.5029) -> (-3.5858, -24.6493) centre (-3.2322, -25.0029) ccw
  line L113 (-3.2322, -24.5029) -> (-0.9536, -24.5029)
  line L114 (7.1142, -25.8564) -> (4.7214, -23.4637)
  line L115 (6, -27.2707) -> (6, -28.0029)
  arc A112 (6, -27.2707) -> (5.8536, -26.9171) centre (5.5, -27.2707) ccw
  line L116 (3.5858, -24.6493) -> (5.8536, -26.9171)
  arc A113 (7.1142, -25.8564) -> (7.4678, -26.0029) centre (7.4678, -25.5029) ccw
  line L117 (8, -26.0029) -> (7.4678, -26.0029)
  arc A114 (8, -26.0029) -> (8.5, -25.5029) centre (8, -25.5029) ccw
  line L118 (8.5, -23.5029) -> (8.5, -25.5029)
  arc A115 (9, -23.0029) -> (8.5, -23.5029) centre (9, -23.5029) ccw
  line L119 (9.3, -23.0029) -> (9, -23.0029)
  arc A116 (9.5, -23.2029) -> (9.3, -23.0029) centre (9.3, -23.2029) ccw
  line L120 (9.5, -23.3029) -> (9.5, -23.2029)
  arc A117 (9.5, -23.3029) -> (9.7, -23.5029) centre (9.7, -23.3029) ccw
  line L121 (9.8, -23.5029) -> (9.7, -23.5029)
  arc A118 (10, -23.7029) -> (9.8, -23.5029) centre (9.8, -23.7029) ccw
  line L122 (10, -28.5029) -> (10, -23.7029)
  arc A119 (-7.4678, -26.0029) -> (-7.1142, -25.8564) centre (-7.4678, -25.5029) ccw
  line L123 (-7.4678, -26.0029) -> (-8, -26.0029)
  arc A120 (-10, -28.5029) -> (-8.5, -30.0029) centre (-8.5, -28.5029) ccw
  arc A121 (-8.5, -25.5029) -> (-8, -26.0029) centre (-8, -25.5029) ccw
  line L124 (-10, -23.7529) -> (-10, -28.5029)
  line L125 (-8.5, -25.5029) -> (-8.5, -23.5029)
  arc A122 (-3, -29.0029) -> (-3.5, -28.5029) centre (-3.5, -29.0029) ccw
  line L126 (-3, -29.3029) -> (-3, -29.0029)
  arc A123 (-3.2, -29.5029) -> (-3, -29.3029) centre (-3.2, -29.3029) ccw
  line L127 (-3.35, -29.5029) -> (-3.2, -29.5029)
  arc A124 (-3.35, -29.5029) -> (-3.55, -29.7029) centre (-3.35, -29.7029) ccw
  line L128 (-3.55, -29.8029) -> (-3.55, -29.7029)
  arc A125 (-3.75, -30.0029) -> (-3.55, -29.8029) centre (-3.75, -29.8029) ccw
  line L129 (-8.5, -30.0029) -> (-3.75, -30.0029)
  line L130 (-3.5, -28.5029) -> (-5.5, -28.5029)
  line L131 (3.55, -29.7029) -> (3.55, -29.8029)
  line L132 (3.2, -29.5029) -> (3.35, -29.5029)
  line L133 (3, -29.0029) -> (3, -29.3029)
  arc A126 (3.55, -29.7029) -> (3.35, -29.5029) centre (3.35, -29.7029) ccw
  arc A127 (3.55, -29.8029) -> (3.75, -30.0029) centre (3.75, -29.8029) ccw
  arc A128 (3, -29.3029) -> (3.2, -29.5029) centre (3.2, -29.3029) ccw
  arc A129 (3.5, -28.5029) -> (3, -29.0029) centre (3.5, -29.0029) ccw
  arc A130 (8.5, -30.0029) -> (10, -28.5029) centre (8.5, -28.5029) ccw
  line L134 (3.75, -30.0029) -> (8.5, -30.0029)
  line L135 (5.5, -28.5029) -> (3.5, -28.5029)
  arc A131 (5.5, -28.5029) -> (6, -28.0029) centre (5.5, -28.0029) ccw
  point P0 (0, 0)
  point P1 (-10, 0)
  constraints: 1 horizontal alignment, 2 other
extrude "Extrusion1" add sketch "Sketch1" along normal mid plane 304.8
body "Solid1"
